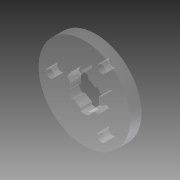
# Autodesk Inventor part: Small Gear Spacer
Saved by Autodesk Inventor 2014 SP1 (Build 180222100, 222)
## iProperties
Created: 2012-03-30
Part Number: Small Gear Spacer
Material: Polycarbonate, Clear
Document SubType Name: Modeling
Designer: Moses
Mass: 13.1156 g
Surface Area: 52.0047 cm^2
Volume: 10.9297 cm^3
Density: 1.2 g/cm^3
Appearance: Polycarbonate - Clear
Author: Moses
Autodesk Inventor part; units mm, degrees
ref_plane "YZ Plane" through (0, 0, 0) normal (1, 0, 0) x (0, 1, 0)
ref_plane "XZ Plane" through (0, 0, 0) normal (0, 1, 0) x (-1, 0, 0)
ref_plane "XY Plane" through (0, 0, 0) normal (0, 0, 1) x (1, 0, 0)
sketch "Sketch1" plane through (0, 0, 0) normal (0, 0, 1) x (1, 0, 0)
  circle A0 centre (0, 0) radius 25.4
  circle A1 centre (-19.05, 0) radius 2.3495
  circle A2 centre (9.525, -16.4978) radius 2.3495
  circle A3 centre (9.525, 16.4978) radius 2.3495
  line L0 (-19.05, 0) -> (0, 0) construction
  dimension "d0" = 50.8
  dimension "d3" = 4.699
  dimension "d6" = 360
  dimension "d8" = 19.05
  constraints: 4 centre point, 2 end point, 1 coincident, 1 horizontal, 7 other
  measures "d0" diameter of A0
  measures "d3" diameter of A1
  measures "d8" distance of L0.start L0.end
extrude "Extrusion1" add sketch "Sketch1" along normal blind 6.35
sketch "Sketch2" plane through (0, 0, 6.35) normal (0, 0, 1) x (1, 0, 0)
  arc A0 (2, 7.9524) -> (-2, 7.9524) centre (0, 0) ccw projected
  arc A1 (-2, 7.9524) -> (-5.8869, 5.7082) centre (0, 0) ccw projected
  arc A2 (-5.8869, 5.7082) -> (-7.8869, 2.2441) centre (0, 0) ccw projected
  arc A3 (-7.8869, 2.2441) -> (-7.8869, -2.2441) centre (0, 0) ccw projected
  arc A4 (-7.8869, -2.2441) -> (-5.8869, -5.7082) centre (0, 0) ccw projected
  arc A5 (-5.8869, -5.7082) -> (-2, -7.9524) centre (0, 0) ccw projected
  arc A6 (-2, -7.9524) -> (2, -7.9524) centre (0, 0) ccw projected
  arc A7 (2, -7.9524) -> (5.8869, -5.7082) centre (0, 0) ccw projected
  arc A8 (5.8869, -5.7082) -> (7.8869, -2.2441) centre (0, 0) ccw projected
  arc A9 (7.8869, -2.2441) -> (7.8869, 2.2441) centre (0, 0) ccw projected
  arc A10 (7.8869, 2.2441) -> (5.8869, 5.7082) centre (0, 0) ccw projected
  arc A11 (5.8869, 5.7082) -> (2, 7.9524) centre (0, 0) ccw projected
  arc A12 (2, 9.7469) -> (-2, 9.7469) centre (0, 0) ccw projected
  line L0 (2, 7.9524) -> (2, 9.7469) projected
  line L1 (-2, 9.7469) -> (-2, 7.9524) projected
  line L2 (-5.8869, 5.7082) -> (-7.4411, 6.6055) projected
  arc A13 (-7.4411, 6.6055) -> (-9.4411, 3.1414) centre (0, 0) ccw projected
  line L3 (-9.4411, 3.1414) -> (-7.8869, 2.2441) projected
  line L4 (-7.8869, -2.2441) -> (-9.4411, -3.1414) projected
  arc A14 (-9.4411, -3.1414) -> (-7.4411, -6.6055) centre (0, 0) ccw projected
  line L5 (-7.4411, -6.6055) -> (-5.8869, -5.7082) projected
  line L6 (-2, -7.9524) -> (-2, -9.7469) projected
  arc A15 (-2, -9.7469) -> (2, -9.7469) centre (0, 0) ccw projected
  line L7 (2, -9.7469) -> (2, -7.9524) projected
  line L8 (5.8869, -5.7082) -> (7.4411, -6.6055) projected
  arc A16 (7.4411, -6.6055) -> (9.4411, -3.1414) centre (0, 0) ccw projected
  line L9 (9.4411, -3.1414) -> (7.8869, -2.2441) projected
  line L10 (7.8869, 2.2441) -> (9.4411, 3.1414) projected
  arc A17 (9.4411, 3.1414) -> (7.4411, 6.6055) centre (0, 0) ccw projected
  line L11 (7.4411, 6.6055) -> (5.8869, 5.7082) projected
extrude "Extrusion2" cut sketch "Sketch2" against normal blind 25.4
body "Solid1"
